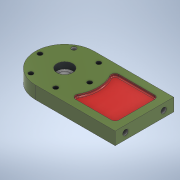
# Autodesk Inventor part: bearing stand without hole
Saved by Autodesk Inventor 2020 (Build 240168000, 168)
## iProperties
Created: 2020-08-08
Part Number: bearing stand without hole
Material: Generic
Document SubType Name: Modeling
Designer: benny
Density: 1 g/cm^3
Appearance: Default
Author: benny
Autodesk Inventor part; units mm, degrees
ref_plane "YZ Plane" through (0, 0, 0) normal (1, 0, 0) x (0, 1, 0)
ref_plane "XZ Plane" through (0, 0, 0) normal (0, 1, 0) x (-1, 0, 0)
ref_plane "XY Plane" through (0, 0, 0) normal (0, 0, 1) x (1, 0, 0)
sketch "Sketch1" plane through (0, 0, 0) normal (0, 1, 0) x (-1, 0, 0)
  line L0 (0, 0) -> (0, -46)
  line L1 (0, -46) -> (125, -46)
  line L2 (125, -46) -> (125, 46)
  line L3 (125, 46) -> (0, 46)
  line L4 (0, 46) -> (0, 0)
  circle A0 centre (125, 0) radius 46
  dimension "d0" = 46
  dimension "d1" = 125
  dimension "d2" = 92
  dimension "d3" = 125
  dimension "d4" = 92
  constraints: 10 end point, 2 perpendicular, 1 centre point, 1 midpoint, 1 point on line, 1 vertical
  measures "d0" distance of L0.start L0.end
  measures "d1" distance of L0.end L1.end
  measures "d2" distance of L1.end L2.end
  measures "d3" distance of L2.end L3.end
  measures "d4" diameter of A0
extrude "Extrusion1" add sketch "Sketch1" along normal blind 20
sketch "Sketch2" plane through (0, 20, 0) normal (0, 1, 0) x (1, 0, 0)
  circle A0 centre (-125, 0) radius 52
  line L0 (-12, 0) -> (-12, 34)
  line L1 (-12, 34) -> (-121.2889, 34)
  line L2 (-121.2889, 34) -> (-121.2889, -34)
  line L3 (-121.2889, -34) -> (-12, -34)
  line L4 (-12, -34) -> (-12, 0)
  point P0 (0, 0)
  point P1 (-85.6554, 34)
  point P2 (-85.6554, -34)
  dimension "d7" = 104
  dimension "d8" = 34
  dimension "d9" = 68
  constraints: 10 end point, 4 perpendicular, 1 centre point, 1 point on line, 1 vertical
  measures "d7" diameter of A0
  measures "d8" distance of L0.start L0.end
  measures "d9" distance of L1.end L2.end
extrude "Extrusion2" cut sketch "Sketch2" against normal blind 4 contours A0 L1 L0 L4 L3
fillet "Fillet1" radius 6 4 edges at (-85.6554, 18, -34) (-85.6554, 18, 34) (-12, 18, 34) (-12, 18, -34)
fillet "Fillet2" radius 2 8 edges at (-79.3725, 16, -31.0513) (-46.1031, 16, -34) (-13.7574, 16, -32.2426) (-12, 16, 0) (-13.7574, 16, 32.2426) (-46.1031, 16, 34) (-79.3725, 16, 31.0513) (-73, 16, 0)
ref_plane "Work Plane1" through (0, 10, 0) normal (0, 1, 0) x (1, 0, 0)
mirror "Mirror1" about plane through (0, 10, 0) normal (0, 1, 0) of "Extrusion2", "Fillet1", "Fillet2"
sketch "Sketch3" plane through (0, 20, 0) normal (0, 1, 0) x (1, 0, 0)
  line L0 (-125, 0) -> (-164, 0)
  circle A0 centre (-164, 0) radius 3.5
  point P0 (0, 0)
  dimension "d15" = 39
  dimension "d16" = 7
  constraints: 2 end point, 1 centre point, 1 coincident, 1 horizontal
  measures "d15" distance of L0.start L0.end
  measures "d16" diameter of A0
extrude "Extrusion3" cut sketch "Sketch3" against normal blind 14
sketch "Sketch4" plane through (0, 0, 0) normal (0, -1, 0) x (1, 0, 0)
  circle A0 centre (-164, 0) radius 6
  point P0 (0, 0)
  dimension "d19" = 12
  constraints: 1 centre point
  measures "d19" diameter of A0
extrude "Extrusion4" cut sketch "Sketch4" against normal blind 6
sketch "Sketch5" plane through (0, 0, 0) normal (0, -1, 0) x (1, 0, 0)
  circle A0 centre (-125, 0) radius 8
  point P0 (0, 0)
  dimension "d22" = 16
  constraints: 1 centre point
  measures "d22" diameter of A0
extrude "Extrusion5" cut sketch "Sketch5" against normal blind 10
sketch "Sketch6" plane through (0, 20, 0) normal (0, 1, 0) x (1, 0, 0)
  circle A0 centre (-125, 0) radius 12.5
  point P0 (0, 0)
  dimension "d25" = 25
  constraints: 1 centre point
  measures "d25" diameter of A0
extrude "Extrusion6" cut sketch "Sketch6" against normal blind 10
pattern_circular "Circular Pattern1" count 6 over 360 about axis through (-125, 20, 0) along (0, -1, 0) of "Extrusion3", "Extrusion4"
sketch "Sketch7" plane through (0, 0, 46) normal (1, 0, 0) x (0, 0, -1)
  line L0 (76, 10) -> (109.9347, 11.3291)
  point P0 (46, 0)
  constraints: 2 end point
hole "Hole1" at (0, 10, -30) direction (-1, 0, 0) diameter 8.376 depth 20 tip angle 118 thread size "M10x1.5" class "6H" standard "ISO Metric profile"
mirror "Mirror2" about plane through (0, 0, 0) normal (0, 0, 1) of "Hole1"
body "Solid1"
